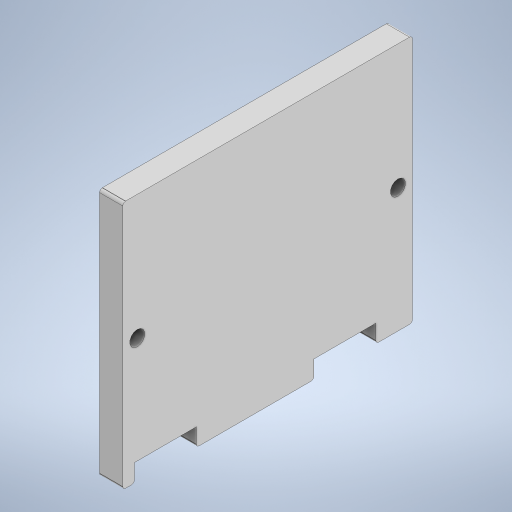
# Autodesk Inventor part: pokrywa
Saved by Autodesk Inventor 2023.5 (Build 275446000, 446)
## iProperties
Created: 2025-04-01
Part Number: pokrywa
Material: Ogólny
Document SubType Name: Modeling
Designer: kamil
Density: 1 g/cm^3
Appearance: Domyślna
Author: kamil
Autodesk Inventor part; units mm, degrees
ref_plane "YZ Plane" through (0, 0, 0) normal (1, 0, 0) x (0, 1, 0)
ref_plane "XZ Plane" through (0, 0, 0) normal (0, 1, 0) x (-1, 0, 0)
ref_plane "XY Plane" through (0, 0, 0) normal (0, 0, 1) x (1, 0, 0)
sketch "Szkic1" plane through (0, 0, 0) normal (1, 0, 0) x (0, 1, 0)
  line L0 (10.7442, -21.3655) -> (23.7442, -21.3655)
  line L1 (23.7442, -21.3655) -> (23.8098, -21.3634)
  arc A0 (23.8098, -21.3634) -> (24.2442, -20.8655) centre (23.7464, -20.8696) ccw
  line L2 (24.2442, -20.8655) -> (24.2442, 28.1345)
  line L3 (24.2442, 28.1345) -> (24.2421, 28.2)
  arc A1 (24.2421, 28.2) -> (23.7442, 28.6345) centre (23.7483, 28.1367) ccw
  line L4 (23.7442, 28.6345) -> (10.7442, 28.6345)
  line L5 (10.7442, 28.6345) -> (10.6787, 28.6324)
  line L6 (3.7484, 28.6345) -> (-18.1981, 28.6345)
  line L7 (-18.1981, 28.6345) -> (-18.2637, 28.6326)
  arc A2 (-18.2637, 28.6326) -> (-18.6981, 28.1345) centre (-18.2006, 28.139) ccw
  line L8 (-18.6981, 28.1345) -> (-18.6981, 27.1345)
  line L9 (-18.6981, 27.1345) -> (-18.6962, 27.0689)
  arc A3 (-18.6962, 27.0689) -> (-18.1981, 26.6345) centre (-18.2025, 27.1322) ccw
  line L10 (-18.1981, 26.6345) -> (-15.6162, 26.6345)
  line L11 (-15.6162, 26.6345) -> (-15.6162, 15.9345)
  line L12 (-15.6162, 15.9345) -> (-18.2023, 15.9345)
  line L13 (-18.2023, 15.9345) -> (-18.2679, 15.9326)
  arc A4 (-18.2679, 15.9326) -> (-18.7023, 15.4345) centre (-18.2048, 15.439) ccw
  line L14 (-18.7023, 15.4345) -> (-18.7023, -3.8655)
  line L15 (-18.7023, -3.8655) -> (-18.7004, -3.9311)
  arc A5 (-18.7004, -3.9311) -> (-18.2023, -4.3655) centre (-18.2067, -3.8678) ccw
  line L16 (-18.2023, -4.3655) -> (-15.6162, -4.3655)
  line L17 (-15.6162, -4.3655) -> (-15.6162, -15.0655)
  line L18 (-15.6162, -15.0655) -> (-18.2023, -15.0655)
  line L19 (-18.2023, -15.0655) -> (-18.2679, -15.0674)
  arc A6 (-18.2679, -15.0674) -> (-18.7023, -15.5655) centre (-18.2048, -15.561) ccw
  line L20 (-18.7023, -15.5655) -> (-18.7023, -20.8655)
  line L21 (-18.7023, -20.8655) -> (-18.7004, -20.9311)
  arc A7 (-18.7004, -20.9311) -> (-18.2023, -21.3655) centre (-18.2067, -20.8678) ccw
  line L22 (-18.2023, -21.3655) -> (3.7442, -21.3655)
  line L23 (3.7442, -21.3655) -> (3.8621, -21.3632)
  circle A8 centre (2.7442, 26.1345) radius 1.3
  circle A9 centre (2.7442, -18.8655) radius 1.3
  line L24 (10.7442, 28.6345) -> (3.7484, 28.6345)
  line L25 (3.7442, -21.3655) -> (10.7442, -21.3655)
  point P0 (0, 0)
  constraints: 52 end point, 16 point on circle, 10 centre point, 10 horizontal, 6 vertical, 1 parallel, 65 other
extrude "Wyciągnięcie proste1" add sketch "Szkic1" along normal blind 4
